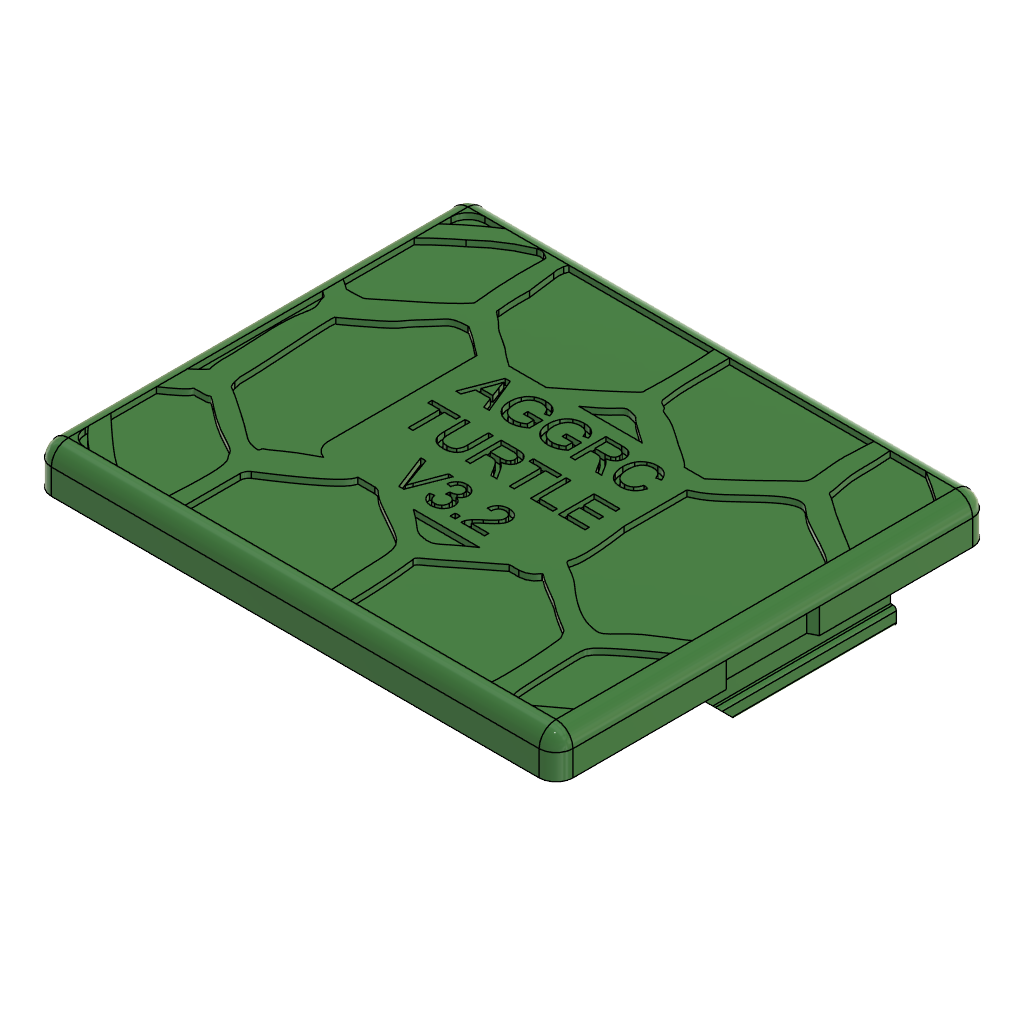
TURTLE_Case_TopV3 (Autodesk Fusion 360 design; units mm, degrees)
Autodesk Fusion 360 part; units mm, degrees
(part 1 of 2)
sketch "Sketch1" plane through (0, 0, 0) normal (0, 0, 1) x (1, 0, 0)
  line L0 (19.1, 22.9) -> (-19.1, 22.9) construction
  line L1 (-19.1, 22.9) -> (-19.1, -22.9) construction
  line L2 (19.1, -22.9) -> (19.1, 22.9) construction
  line L3 (19.1, 22.9) -> (-19.1, -22.9) construction
  line L4 (-19.1, 22.9) -> (19.1, -22.9) construction
  line L5 (18.1, -21.701) -> (18.1, -21.7) construction
  circle A0 centre (16.3, -20.1) radius 1.8 construction
  circle A1 centre (-16.3, -20.1) radius 1.8 construction
  line L6 (-7.8453, -9.4062) -> (-6.5, -9.4062) construction
  line L7 (-19.1, -22.9) -> (19.1, -22.9) construction
  line L8 (7.3, -22.9) -> (0.3, -22.9) construction
  line L9 (0.3, -22.9) -> (0.3, -10.4809) construction
  line L10 (0.3, -10.4809) -> (7.3, -10.4809) construction
  line L11 (7.3, -10.4809) -> (7.3, -22.9) construction
  line L12 (-11.4, -22.9) -> (-4.4, -22.9) construction
  line L13 (-4.4, -22.9) -> (-4.4, -10.4508) construction
  line L14 (-4.4, -10.4508) -> (-11.4, -10.4508) construction
  line L15 (-11.4, -10.4508) -> (-11.4, -22.9) construction
  line L16 (20.1, 22.9) -> (20.1, 23.7) construction
  line L17 (25.2, 25.2) -> (32.7, 25.2) construction
  line L18 (32.7, 25.2) -> (25.2, 25.2) construction
  line L19 (25.2, 25.2) -> (25.2, 16) construction
  line L20 (25.2, 16) -> (32.7, 16) construction
  line L21 (32.7, 16) -> (32.7, 25.2) construction
  line L22 (32.7, 25.2) -> (32.7, 23.7) construction
  line L23 (32.7, 23.7) -> (37.9, 23.7) construction
  line L24 (37.9, 23.7) -> (20.1, 23.7) construction
  line L25 (20.1, 23.7) -> (20.1, -19.5) construction
  line L26 (37.9, -19.5) -> (37.9, 23.7) construction
  line L27 (37.9, 23.7) -> (-19.1, 23.7) construction
  line L28 (-19.1, 23.7) -> (-19.1, -22.9) construction
  line L29 (-19.1, -22.9) -> (37.9, -22.9) construction
  line L30 (37.9, -22.9) -> (37.9, 23.7) construction
  line L31 (38.3, 24.1) -> (-19.5, 24.1) construction
  line L32 (-19.5, 24.1) -> (-19.5, -23.3) construction
  line L33 (-19.5, -23.3) -> (38.3, -23.3) construction
  line L34 (38.3, -23.3) -> (38.3, 24.1) construction
  line L35 (-19.5, 24.1) -> (38.3, 24.1)
  line L36 (38.3, 24.1) -> (38.3, -23.3)
  line L37 (38.3, -23.3) -> (-19.5, -23.3)
  line L38 (-19.5, -23.3) -> (-19.5, 24.1)
  line L39 (19.1, 22.9) -> (19.3, 22.9) construction
  line L40 (20.1, 22.9) -> (19.9, 22.9) construction
  line L41 (19.9, 23.7) -> (19.9, -23.3)
  line L42 (19.9, -23.3) -> (19.3, -23.3)
  line L43 (19.3, -23.3) -> (19.3, 23.7)
  line L44 (19.3, 23.7) -> (19.3, 24.1)
  line L45 (19.9, 23.7) -> (19.9, 24.1)
  circle A2 centre (-16.3, -20.1) radius 1.5
  circle A3 centre (16.3, -20.1) radius 1.5
  line L46 (25.2, 25.2) -> (25.2, 16) construction
  line L47 (16.7646, 20.1) -> (16.798, 20.1) construction
  circle A4 centre (16.6536, 20.4536) radius 1.5
  circle A5 centre (-16.5121, 20.3121) radius 1.5
  arc A6 (-17.5728, 21.3728) -> (-17.7041, 21.2263) centre (-16.3, 20.1) ccw construction
  line L48 (38.3, -19.9) -> (38.3, -19.4) construction
  line L49 (-14.9395, -20.1) -> (-14.9395, -20.6)
  line L50 (-14.9395, -20.1) -> (14.9498, -20.1)
  line L51 (14.9498, -20.1) -> (14.9498, -23.3)
  line L52 (14.9498, -23.3) -> (-14.9395, -23.3)
  line L53 (-14.9395, -23.3) -> (-14.9395, -20.1)
  line L54 (-14.9395, -20.6) -> (-14.5708, -20.6)
  line L55 (14.9498, -20.6) -> (14.9503, -20.6)
  line L56 (40.2, -25.2) -> (-21.4, -25.2)
  line L57 (-21.4, -25.2) -> (-21.4, 26)
  line L58 (-21.4, 26) -> (40.2, 26)
  line L59 (40.2, 26) -> (40.2, -25.2)
  line L60 (41.2, -26.2) -> (-22.4, -26.2)
  line L61 (-22.4, -26.2) -> (-22.4, 27)
  line L62 (-22.4, 27) -> (41.2, 27)
  line L63 (41.2, 27) -> (41.2, -26.2)
  line L64 (32.7, 24.0729) -> (25.2, 24.0729)
  line L65 (25.2, 24.0729) -> (25.2, 18.0729)
  line L66 (25.2, 18.0729) -> (32.7, 18.0729)
  line L67 (32.7, 18.0729) -> (32.7, 24.0729)
  line L68 (38.3, -19.65) -> (19.9, -19.65)
  line L69 (20.1, -19.4989) -> (19.9, -19.5)
  dimension "d1" = 38.2
  dimension "d2" = 45.8
  dimension "d5" = 3.6
  dimension "d7" = 2.8
  dimension "d13" = 7
  dimension "d14" = 11.8
  dimension "d15" = 7
  dimension "d16" = 7.7
  dimension "d17" = 1
  dimension "d23" = 7.5
  dimension "d24" = 9.2
  dimension "d25" = 1.5
  dimension "d26" = 5.2
  dimension "d27" = 17.8
  dimension "d28" = 43.2
  dimension "d31" = 0.4
  dimension "d36" = 0.2
  dimension "d37" = 0.2
  dimension "d54" = 3
  dimension "d57" = 3
  dimension "d67" = 3
  dimension "d69" = 0.3
  dimension "d70" = 3
  dimension "d89" = 0.5
  dimension "d237" = -1
  dimension "d283" = 6
  constraint horizontal L0
  constraint perpendicular L0 L1
  constraint parallel L1 L2
  constraint coincident L3 origin
  constraint coincident L4 origin
  constraint coincident L4 L5.start
  constraint horizontal L6
  constraint coincident L3 L6.start
  constraint perpendicular L2 L7
  constraint horizontal L8
  constraint vertical L9
  constraint horizontal L10
  constraint vertical L11
  constraint coincident L7 L8.start
  constraint horizontal L12
  constraint vertical L13
  constraint horizontal L14
  constraint vertical L15
  constraint coincident L7 L12.start
  constraint perpendicular L16 L17
  constraint horizontal L18
  constraint vertical L19
  constraint horizontal L20
  constraint vertical L21
  constraint perpendicular L17 L22
  constraint perpendicular L22 L23
  constraint horizontal L24
  constraint vertical L25
  constraint vertical L26
  constraint horizontal L27
  constraint vertical L28
  constraint horizontal L29
  constraint vertical L30
  constraint horizontal L35
  constraint vertical L36
  constraint horizontal L37
  constraint vertical L38
  constraint perpendicular L2 L39
  constraint perpendicular L16 L40
  constraint vertical L41
  constraint horizontal L42
  constraint vertical L43
  constraint coincident L37 L41.end
  constraint coincident L27 L43.end
  constraint coincident L35 L44.end
  constraint perpendicular L35 L44
  constraint coincident L31 L45.end
  constraint perpendicular L31 L45
  constraint concentric A0 A3
  constraint perpendicular L24 L46
  constraint coincident L34 L48.start
  constraint horizontal L47
  constraint coincident L3 L47.start
  constraint coincident A5 A6.start
  constraint coincident L4 A6.end
  constraint coincident L41 L69.end
  constraint perpendicular L49 L54
  constraint horizontal L50
  constraint vertical L51
  constraint horizontal L52
  constraint vertical L53
  constraint coincident L33 L51.end
  constraint coincident L51 L55.start
  constraint collinear L54 L55
  constraint coincident A1 L54.end
  constraint horizontal L64
  constraint vertical L65
  constraint horizontal L66
  constraint vertical L67
  constraint coincident L21 L64.start
  constraint midpoint L48 L68.start
  constraint coincident L41 L68.end
  constraint perpendicular L41 L68
  constraint coincident L25 L69.start
  measures "d1" distance of L1.end L2.start
  measures "d2" distance of L0.end L1.end
  measures "d5" diameter of A0
  measures "d7" distance of L2 A0.centre
  measures "d13" distance of L8.start L8.end
  measures "d14" distance of L2 L11
  measures "d15" distance of L12.start L12.end
  measures "d16" distance of L1 L15
  measures "d17" distance of L0.start L16.start
  measures "d23" distance of L17.end L17.start
  measures "d24" distance of L17.end L20.end
  measures "d25" distance of L17.end L22.end
  measures "d26" distance of L22.end L23.end
  measures "d27" distance of L23.end L16.end
  measures "d28" distance of L23.end L26.start
  measures "d36" distance of L0.start L39.end
  measures "d37" distance of L16.start L40.end
  measures "d54" diameter of A2
  measures "d57" diameter of A3
  measures "d67" diameter of A4
  measures "d69" distance of A6.centre A5.centre
  measures "d70" diameter of A5
  measures "d89" distance of L48.start L48.end
  measures "d283" distance of L64.start L66.end
extrude "Extrude1" add sketch "Sketch1" along normal blind 2 contours L35 L37 L38 L43 L44 A2 A3 L50 L51 L53 | L35 L37 L41 L42 L43 L44 L45 | L35 L36 L41 L45 L68 | L64 L65 L66 L67 makes body 1
extrude "Extrude2" add sketch "Sketch1" along normal blind 10.2 contours L36 L37 L41 L68 | L56 L57 L58 L59 bodies 1
extrude "Extrude16" add sketch "Sketch1" along normal blind 6 contours L37 A2 A3 L50 L51 L52 L53 bodies 1
extrude "Extrude3" add sketch "Sketch1" along normal blind 10 contours A2 L53 L54 | A2 L49 L50 L53 | A3 L50 L51 | A3 L50 L51 | A2 L49 L50 L53 L54 | A4 | A5 bodies 1
extrude "Extrude12" add sketch "Sketch1" along normal blind 16 contours L35 L37 L41 L42 L43 L44 L45 bodies 1
extrude "Extrude32" add sketch "Sketch1" along normal blind 6 contours L64 L65 L66 L67 bodies 1
ref_plane "WorkPlane1" through (9.4, 0.4, 10.2) normal (0, 0, 1) x (1, 0, 0)
sketch "Sketch3" plane through (0, 0, 10.2) normal (0, 0, 1) x (1, 0, 0)
  line L0 (25.2, 25.2) -> (25.2, 16)
  line L1 (32.7, 25.2) -> (25.2, 25.2)
  line L2 (32.7, 16) -> (32.7, 25.2)
  line L3 (25.2, 16) -> (32.7, 16)
  line L4 (25.2, 24.1) -> (24.9, 24.1) construction
  line L5 (32.7, 24.1) -> (33, 24.1) construction
  line L6 (24.9, 24.1) -> (33, 24.1)
  line L7 (33, 24.1) -> (33, 26)
  line L8 (24.9, 26) -> (24.9, 24.1)
  line L9 (0.3, -22.9) -> (0.3, -10.4809)
  line L10 (0.3, -10.4809) -> (7.3, -10.4809)
  line L11 (7.3, -10.4809) -> (7.3, -22.9)
  line L12 (-19.1, -22.9) -> (37.9, -22.9)
  line L13 (-4.4, -22.9) -> (-4.4, -10.4508)
  line L14 (-4.4, -10.4508) -> (-11.4, -10.4508)
  line L15 (-11.4, -10.4508) -> (-11.4, -22.9)
  line L16 (7.3, -22.9) -> (8, -22.9) construction
  line L17 (0.3, -22.9) -> (-0.4, -22.9) construction
  line L18 (-4.4, -22.9) -> (-3.7, -22.9) construction
  line L19 (8, -23.3) -> (8, -22.9)
  line L20 (-12.1, -22.9) -> (-12.1, -25.2)
  line L21 (-3.7, -25.2) -> (-3.7, -23.3)
  line L22 (-19.5, -23.3) -> (-19.5, 24.1)
  line L23 (-19.5, 24.1) -> (38.3, 24.1)
  line L24 (19.9, 23.7) -> (19.9, -23.3)
  line L25 (19.3, -23.3) -> (19.3, 23.7)
  line L26 (19.9, 23.7) -> (19.9, 24.1)
  line L27 (19.3, 23.7) -> (19.3, 24.1)
  line L28 (38.3, -23.3) -> (38.3, 24.1)
  line L29 (-19.5, -23.3) -> (38.3, -23.3)
  line L30 (19.9, -22.9) -> (38.3, -22.9)
  line L31 (38.3, -22.9) -> (38.3, -19.9)
  line L32 (19.9, -19.9) -> (19.9, -22.9)
  line L33 (38.3, 24.1) -> (38.3, -19.65)
  line L34 (19.9, -23.3) -> (19.3, -23.3)
  line L35 (24.9, 24.1) -> (33, 24.1)
  line L36 (33, 24.1) -> (33, 27)
  line L37 (33, 27) -> (24.9, 27)
  line L38 (24.9, 27) -> (24.9, 24.1)
  line L39 (-11.4, -22.9) -> (-3.6915, -22.9)
  line L40 (-3.6915, -26.2) -> (-12.1, -26.2)
  line L41 (-0.4, -22.9) -> (8.0023, -22.9)
  line L42 (8.0023, -23.3) -> (8.0023, -26.2)
  line L43 (8.0023, -26.2) -> (-0.4, -26.2)
  line L44 (-0.4, -26.2) -> (-0.4, -22.9)
  line L45 (-3.6915, -22.9) -> (-3.6915, -23.3)
  line L46 (-3.6915, -25.2) -> (-3.6915, -26.2)
  line L47 (-12.1, -26.2) -> (-12.1, -25.2)
  line L48 (-3.7, -22.9) -> (-4.4, -22.9)
  line L49 (-11.4, -22.9) -> (-12.1, -22.9)
  line L50 (8, -22.9) -> (7.3, -22.9)
  line L51 (0.3, -22.9) -> (-0.4, -22.9)
  line L52 (-3.6915, -22.9) -> (-12.1, -22.9)
  line L53 (-12.1, -22.9) -> (-12.1, -26.2)
  line L54 (-12.1, -26.2) -> (-3.6915, -26.2)
  line L55 (-3.6915, -26.2) -> (-3.6915, -22.9)
  line L56 (19.3, -23.3) -> (-19.5, -23.3)
  line L57 (-19.5, -23.3) -> (-19.5, 24.1)
  line L58 (-19.5, 24.1) -> (19.3, 24.1)
  line L59 (19.3, 24.1) -> (19.9, 24.1)
  line L60 (40.2, 26) -> (-21.4, 26)
  line L61 (-21.4, 26) -> (-21.4, -25.2)
  line L62 (-21.4, -25.2) -> (40.2, -25.2)
  line L63 (40.2, -25.2) -> (40.2, 26)
  line L64 (38.3, -19.65) -> (19.9, -19.65)
  line L65 (19.9, -19.65) -> (19.9, -23.3)
  line L66 (19.9, 24.1) -> (38.3, 24.1)
  dimension "d59" = 0.3
  dimension "d60" = 0.3
  dimension "d71" = 0.7
  dimension "d72" = 0.7
  dimension "d73" = 0.7
  constraint coincident L0 L4.start
  constraint perpendicular L0 L4
  constraint coincident L2 L5.start
  constraint perpendicular L2 L5
  constraint perpendicular L6 L7
  constraint parallel L7 L8
  constraint perpendicular L2 L6
  constraint coincident L11.end L16.start
  constraint perpendicular L11 L16
  constraint coincident L9.start L17.start
  constraint perpendicular L9 L17
  constraint coincident L13.start L18.start
  constraint perpendicular L13 L18
  constraint horizontal L50
  constraint vertical L19
  constraint horizontal L48
  constraint vertical L20
  constraint vertical L21
  constraint horizontal L30
  constraint vertical L31
  constraint vertical L32
  constraint coincident L24 L30.start
  constraint coincident L12 L30.start
  constraint horizontal L35
  constraint vertical L36
  constraint horizontal L37
  constraint vertical L38
  constraint horizontal L39
  constraint vertical L45
  constraint horizontal L40
  constraint vertical L47
  constraint horizontal L41
  constraint vertical L42
  constraint horizontal L43
  constraint vertical L44
  constraint coincident L29 L21.end
  constraint coincident L29 L45.end
  constraint collinear L45 L46
  constraint collinear L48 L49
  constraint collinear L50 L51
  constraint coincident L29 L19.start
  constraint coincident L29 L42.start
  constraint horizontal L52
  constraint vertical L53
  constraint horizontal L54
  constraint vertical L55
  measures "d59" distance of L4.start L4.end
  measures "d60" distance of L5.start L5.end
  measures "d71" distance of L11.end L16.end
  measures "d72" distance of L9.start L17.end
  measures "d73" distance of L13.start L18.end
extrude "Extrude5" cut sketch "Sketch3" against normal blind 3.9 contours L0 L1 L2 L6 L23 L35 L66 | L0 L1 L2 L6 L7 L8 L23 L35 L36 L38 L60 L66 | L36 L37 L38 L60 | L40 L46 L47 L53 L54 L55 L62 | L20 L21 L29 L53 L56 L62 | L29 L42 L44 L56 L62 | L42 L43 L44 L62 | L12 L20 L29 L39 L45 L48 L49 L52 L53 L55 L56 | L21 L29 L55 L56 L62 | L12 L19 L29 L41 L44 L50 L51 L56 bodies 1
extrude "Extrude13" add sketch "Sketch3" along normal blind 14.2 contours L0 L1 L2 L6 L23 L35 L66 | L0 L1 L2 L6 L7 L8 L23 L35 L36 L38 L60 L66 | L8 L20 L22 L23 L29 L38 L53 L56 L57 L58 L59 L60 L61 L62 L66 | L7 L23 L28 L29 L31 L33 L34 L36 L42 L56 L60 L62 L63 L66 | L29 L44 L55 L56 L62 bodies 1
sketch "Sketch10" plane through (0, 0, 24.4) normal (0, 0, 1) x (-1, 0, 0)
  line L0 (19.5, -24.1) -> (-38.3, -24.1)
  line L1 (3.6915, 23.3) -> (12.1, 23.3)
  line L2 (12.1, 23.3) -> (12.1, 25.2)
  line L3 (3.6915, 25.2) -> (3.6915, 23.3)
  line L4 (0.4, 25.2) -> (0.4, 23.3)
  line L5 (0.4, 23.3) -> (3.6915, 23.3)
  line L6 (3.6915, 23.3) -> (3.6915, 25.2)
  line L7 (-8.0023, 23.3) -> (0.4, 23.3)
  line L8 (0.4, 23.3) -> (0.4, 25.2)
  line L9 (-8.0023, 25.2) -> (-8.0023, 23.3)
  line L10 (12.1, 23.3) -> (19.5, 23.3)
  line L11 (19.5, 23.3) -> (19.5, -24.1)
  line L12 (-38.3, -24.1) -> (-38.3, 23.3)
  line L13 (-38.3, 23.3) -> (-8.0023, 23.3)
  line L14 (-8.0023, 23.3) -> (-8.0023, 25.2)
  line L15 (-8.0023, 25.2) -> (-40.2, 25.2)
  line L16 (-40.2, 25.2) -> (-40.2, -26)
  line L17 (-40.2, -26) -> (21.4, -26)
  line L18 (21.4, -26) -> (21.4, 25.2)
  line L19 (21.4, 25.2) -> (12.1, 25.2)
  line L20 (12.1, 25.2) -> (12.1, 23.3)
  line L21 (12.1, 25.2) -> (3.6915, 25.2)
  line L22 (3.6915, 25.2) -> (0.4, 25.2)
  line L23 (0.4, 25.2) -> (-8.0023, 25.2)
extrude "Extrude22" add sketch "Sketch10" along normal blind 7 contours L0 L2 L9 L10 L11 L12 L13 L14 L15 L16 L17 L18 L19 L20 | L1 L2 L3 L6 L20 L21 | L4 L7 L8 L9 L14 L23 | L3 L4 L5 L6 L8 L22 bodies 1
sketch "Sketch13" plane through (0, 0, 31.4) normal (0, 0, 1) x (-1, 0, 0)
  line L0 (-38.3, 23.3) -> (19.5, 23.3)
  line L1 (-7.9258, 23.3) -> (-7.9258, 23.1) construction
  line L2 (-38.3, 23.3) -> (-38.3, -0.4) construction
  line L3 (19.5, 23.3) -> (19.5, -0.4) construction
  line L4 (-38.3, -0.4) -> (-38.3, 17.6) construction
  line L5 (-38.3, -0.4) -> (-38.3, -18.4) construction
  line L6 (19.5, -0.4) -> (19.5, 17.6) construction
  line L7 (19.5, -0.4) -> (19.5, -18.4) construction
  line L8 (19.5, 17.6) -> (18.5, 17.6) construction
  line L9 (19.5, 17.6) -> (18.5, 17.6)
  line L10 (19.5, -18.4) -> (19.3, -18.4)
  line L11 (19.3, -18.4) -> (18.3, -18.4)
  line L12 (18.3, -18.4) -> (19.3, -18.4)
  line L13 (19.3, 17.6) -> (18.3, 17.6)
  line L14 (19.5, 23.3) -> (19.5, -24.1)
  line L15 (19.5, -24.1) -> (-38.3, -24.1)
  line L16 (-38.3, -24.1) -> (-38.3, 23.3)
  line L17 (21.4, 25.2) -> (-40.2, 25.2)
  line L18 (-40.2, 25.2) -> (-40.2, -26)
  line L19 (-40.2, -26) -> (21.4, -26)
  line L20 (21.4, -26) -> (21.4, 25.2)
  line L21 (-37.1, 10.6) -> (-38.1, 10.6) construction
  line L22 (-37.1, -16.4) -> (-37.1, 10.6)
  line L23 (-37.1, 10.6) -> (-38.1, 10.6)
  line L24 (-38.1, 10.6) -> (-38.1, -16.4)
  line L25 (-38.1, -16.4) -> (-37.1, -16.4)
  line L26 (-38.1, -16.4) -> (-38.3, -16.4)
  line L27 (-38.3, -16.4) -> (-38.3, 10.6)
  line L28 (-38.3, 10.6) -> (-38.1, 10.6)
  line L29 (19.3, -18.4) -> (19.5, -18.4)
  line L30 (19.5, -18.4) -> (19.5, 17.6)
  line L31 (19.5, 17.6) -> (19.3, 17.6)
  line L32 (19.3, 17.6) -> (19.3, -18.4)
  line L33 (18.3, 17.6) -> (18.3, -18.4)
  line L34 (19.3, 17.6) -> (19.3, -18.4)
  line L35 (-38.1, -16.4) -> (-38.1, 10.6)
  line L36 (18.3, -22.9) -> (-37.1, -22.9)
  line L37 (-37.1, 22.1) -> (18.3, 22.1)
  line L38 (18.3, 17.6) -> (18.3, -18.4)
  line L39 (19.3, 17.6) -> (19.3, -18.4)
  line L40 (-37.1, -16.4) -> (-37.1, 10.6)
  line L41 (-38.1, -16.4) -> (-38.1, 10.6)
  line L42 (18.3, 22.1) -> (19.5, 22.1)
  line L43 (-37.1, 22.1) -> (-38.3, 22.1)
  line L44 (18.3, -22.9) -> (19.5, -22.9)
  line L45 (-37.1, -22.9) -> (-38.3, -22.9)
  dimension "d189" = 0.2
  dimension "d192" = 23.7
  dimension "d193" = 23.7
  dimension "d194" = 18
  dimension "d195" = 18
  dimension "d196" = 18
  dimension "d197" = 18
  dimension "d199" = 1
  constraint coincident L0 L1.start
  constraint coincident L0.start L2.start
  constraint perpendicular L0 L2
  constraint coincident L0.end L3.start
  constraint perpendicular L0 L3
  constraint parallel L2 L4
  constraint parallel L3 L6
  constraint perpendicular L3 L8
  constraint perpendicular L7 L10
  constraint perpendicular L7 L11
  constraint parallel L12 L13
  constraint perpendicular L22 L23
  constraint parallel L22 L24
  constraint parallel L23 L25
  constraint perpendicular L21 L22
  constraint horizontal L26
  constraint vertical L27
  constraint horizontal L28
  constraint coincident L16 L27.end
  constraint horizontal L29
  constraint vertical L30
  constraint horizontal L31
  constraint vertical L32
  constraint coincident L3 L42.end
  constraint coincident L2 L43.end
  constraint coincident L14 L44.end
  constraint perpendicular L14 L44
  constraint coincident L16 L45.end
  constraint perpendicular L16 L45
  measures "d189" distance of L1.start L1.end
  measures "d192" distance of L0.start L2.end
  measures "d193" distance of L0.end L3.end
  measures "d194" distance of L2.end L4.end
  measures "d195" distance of L2.end L5.end
  measures "d196" distance of L3.end L6.end
  measures "d197" distance of L3.end L7.end
  measures "d199" distance of L6.end L8.end
extrude "Extrude23" add sketch "Sketch13" along normal blind 5 separate body contours L0 L14 L16 L37 L42 L43 | L9 L10 L11 L12 L13 L14 L16 L22 L23 L25 L26 L28 L29 L31 L33 L36 L37 L38 L40 L42 L43 L44 L45 | L16 L24 L26 L27 L28 L35 L41 | L9 L10 L14 L29 L30 L31 L32 L34 L39 | L22 L23 L24 L25 L35 L40 L41 | L9 L11 L12 L13 L32 L33 L34 L38 L39 | L14 L15 L16 L36 L44 L45 | L17 L18 L19 L20 makes body 2
extrude "Extrude25" add sketch "Sketch13" against normal blind 5 contours L22 L23 L24 L25 L35 L40 L41 | L9 L11 L12 L13 L32 L33 L34 L38 L39 bodies 2
ref_plane "WorkPlane2" through (9.4, 0.4, 33.9) normal (1, 0, 0) x (0, 1, 0)
sketch "Sketch19" plane through (38.1, 0, 0) normal (1, 0, 0) x (0, 1, 0)
  line L0 (-10.6, 26.4) -> (16.4, 26.4)
  line L1 (16.4, 26.4) -> (-10.6, 26.4)
  line L2 (-10.6, 26.4) -> (-10.6, 28.4)
  line L3 (-10.6, 28.4) -> (16.4, 28.4)
  line L4 (16.4, 28.4) -> (16.4, 26.4)
  line L5 (16.4, 31.4) -> (-10.6, 31.4)
  line L6 (-10.6, 31.4) -> (-10.6, 26.4)
  line L7 (16.4, 26.4) -> (16.4, 31.4)
  dimension "d269" = 2
  constraint perpendicular L1 L2
  constraint parallel L1 L3
  constraint parallel L2 L4
  constraint coincident L0.start L1.end
  constraint coincident L0.end L1.start
  measures "d269" distance of L0.end L3.end
sketch "Sketch26" plane through (-19.3, 0, 0) normal (-1, 0, 0) x (0, -1, 0)
  line L0 (17.6, 31.4) -> (-18.4, 31.4)
  line L1 (-18.4, 31.4) -> (-18.4, 26.4)
  line L2 (-18.4, 26.4) -> (17.6, 26.4)
  line L3 (17.6, 26.4) -> (17.6, 31.4)
  line L4 (17.6, 26.4) -> (-18.4023, 26.4)
  line L5 (-18.4023, 26.4) -> (-18.4023, 28.4)
  line L6 (-18.4023, 28.4) -> (17.6, 28.4)
  line L7 (17.6, 28.4) -> (17.6, 26.4)
  dimension "d327" = 2
  constraint horizontal L4
  constraint vertical L5
  constraint horizontal L6
  constraint vertical L7
  constraint coincident L2.end L3.start
  measures "d327" distance of L2.end L6.end
extrude "Extrude27" add sketch "Sketch26" along normal blind 0.7 contours L1 L2 L3 L4 L6 L7 bodies 2
extrude "Extrude31" add sketch "Sketch19" along normal blind 0.7 contours L0 L1 L2 L3 L4 L6 L7 bodies 2
sketch "Sketch18" plane through (40.2, 0, 0) normal (1, 0, 0) x (0, 1, 0)
  line L0 (-25.2, 31.4) -> (26, 31.4)
  line L1 (26, 31.4) -> (26, 36.4)
  line L2 (26, 36.4) -> (-25.2, 36.4)
  line L3 (-25.2, 36.4) -> (-25.2, 31.4)
  line L4 (-25.2, 31.4) -> (0.4, 31.4) construction
  line L5 (0.4, 31.4) -> (5.4, 31.4) construction
  line L6 (0.4, 31.4) -> (-4.6, 31.4) construction
  line L7 (-4.6, 31.4) -> (5.4, 31.4)
  line L8 (5.4, 31.4) -> (5.4, 33.9)
  line L9 (5.4, 33.9) -> (-4.6, 33.9)
  line L10 (-4.6, 33.9) -> (-4.6, 31.4)
  dimension "d257" = 25.6
  dimension "d258" = 5
  dimension "d259" = 5
  dimension "d260" = 10
  dimension "d261" = 2.5
  constraint coincident L0.start L3.end
  constraint perpendicular L3 L4
  constraint coincident L0 L5.end
  constraint parallel L4 L6
  constraint horizontal L7
  constraint vertical L8
  constraint horizontal L9
  constraint vertical L10
  measures "d257" distance of L0.start L4.end
  measures "d258" distance of L4.end L5.end
  measures "d259" distance of L4.end L6.end
  measures "d260" distance of L6.end L5.end
  measures "d261" distance of L6.end L9.end
extrude "Extrude30" cut sketch "Sketch18" against normal blind 1 contours L0 L7 L8 L9 L10 bodies 2
mirror "Mirror2" about plane through (9.4, 0.4, 33.9) normal (1, 0, 0) of "Extrude30"
sketch "Sketch16" plane through (-19.5, 0, 0) normal (1, 0, 0) x (0, 1, 0)
  line L0 (-23.3, 2) -> (24.1, 2)
  line L1 (24.1, 2) -> (24.1, 31.4)
  line L2 (24.1, 31.4) -> (-23.3, 31.4)
  line L3 (-23.3, 31.4) -> (-23.3, 2)
  line L4 (-23.3, 31.4) -> (0.4, 31.4) construction
  line L5 (0.4, 31.4) -> (0.4, 28.4) construction
  line L6 (0.4, 28.4) -> (0.4, 26.4) construction
  line L7 (0.4, 26.4) -> (18.4, 26.4) construction
  line L8 (0.4, 26.4) -> (-17.6, 26.4) construction
  line L9 (-17.6, 26.4) -> (-17.6, 28.4) construction
  line L10 (-17.6, 28.4) -> (-17.6, 26.4)
  line L11 (-17.6, 26.4) -> (18.4, 26.4)
  line L12 (18.4, 26.4) -> (18.4, 28.4)
  line L13 (18.4, 28.4) -> (-17.6, 28.4)
  dimension "d222" = 23.7
  dimension "d223" = 3
  dimension "d224" = 2
  dimension "d225" = 18
  dimension "d226" = 18
  dimension "d227" = 2
  constraint coincident L2.end L3.start
  constraint midpoint L2 L4.end
  constraint perpendicular L4 L5
  constraint perpendicular L2 L6
  constraint perpendicular L6 L7
  constraint perpendicular L6 L8
  constraint perpendicular L8 L9
  constraint perpendicular L10 L11
  constraint parallel L10 L12
  constraint parallel L11 L13
  measures "d222" distance of L2.end L4.end
  measures "d223" distance of L4.end L5.end
  measures "d224" distance of L5.end L6.end
  measures "d225" distance of L6.end L7.end
  measures "d226" distance of L6.end L8.end
  measures "d227" distance of L8.end L9.end
extrude "Extrude28" cut sketch "Sketch16" against normal blind 0.7 contours L10 L11 L12 L13 bodies 1
extrude "Extrude29" cut sketch "Sketch13" along normal blind 3 contours L9 L10 L11 L12 L13 L14 L16 L22 L23 L25 L26 L28 L29 L31 L33 L36 L37 L38 L40 L42 L43 L44 L45 | L9 L10 L14 L29 L30 L31 L32 L34 L39 bodies 2
extrude "Extrude35" add sketch "Sketch13" against normal blind 2 contours L0 L14 L16 L37 L42 L43 | L14 L15 L16 L36 L44 L45 bodies 2
mirror "Mirror3" about plane through (9.4, 0.4, 33.9) normal (1, 0, 0) of "Extrude28"
sketch "Sketch17" plane through (9.4, 0, 0) normal (1, 0, 0) x (0, 1, 0)
fillet "Fillet16" radius 2 8 edges at (40.2, -25.2, 15.7) (40.2, 26, 15.7) (-21.4, 26, 15.7) (-21.4, -25.2, 15.7) (40.2, -25.2, 33.9) (40.2, 26, 33.9) (-21.4, 26, 33.9) (-21.4, -25.2, 33.9) on bodies 1 2
sketch "Sketch24" plane through (0, 0, 36.4) normal (0, 0, 1) x (-1, 0, 0)
  arc A0 (21.4, 23.2) -> (19.4, 25.2) centre (19.4, 23.2) ccw
  line L0 (19.4, 25.2) -> (-38.2, 25.2)
  arc A1 (-38.2, 25.2) -> (-40.2, 23.2) centre (-38.2, 23.2) ccw
  line L1 (-40.2, 23.2) -> (-40.2, -24)
  arc A2 (-40.2, -24) -> (-38.2, -26) centre (-38.2, -24) ccw
  line L2 (-38.2, -26) -> (19.4, -26)
  arc A3 (19.4, -26) -> (21.4, -24) centre (19.4, -24) ccw
  line L3 (21.4, -24) -> (21.4, 23.2)
  arc A4 (11.3811, -26) -> (21.4, -18.5141) centre (-2.7859, 3.4081) ccw
  arc A5 (11.0665, -23.7947) -> (16.1393, -20.5124) centre (4.942, -8.7683) ccw
  arc A6 (16.1393, -20.5124) -> (21.4, -15.4127) centre (-2.5631, 4.0438) ccw
  arc A7 (21.4, -15.4127) -> (21.4062, -15.4048) centre (-2.7344, 3.4965) ccw
  arc A8 (8.8605, -25.5305) -> (10.472, -26) centre (19.6633, 8.5476) ccw
  arc A9 (8.8605, -25.5305) -> (8.7, -26) centre (25.0805, -31.338) ccw
  arc A10 (9.6, -23.4) -> (10.2246, -23.7543) centre (15.2927, -14.0914) ccw
  arc A11 (9.534, -23.0852) -> (9.6, -23.4) centre (10.4467, -23.0583) ccw
  arc A12 (9.534, -23.0852) -> (9.2, -14.6) centre (-44.1135, -20.948) ccw
  arc A13 (6.7, -26) -> (7.63, -23.5408) centre (-18.1541, -15.1955) ccw
  arc A14 (7.63, -23.5408) -> (7.6141, -22.3338) centre (4.9418, -22.9727) ccw
  arc A15 (7.6141, -22.3338) -> (7.1948, -19.0652) centre (-155.4891, -41.592) ccw
  arc A16 (7.1948, -19.0652) -> (7.051, -15.2896) centre (-16.615, -18.0816) ccw
  spline S0 degree 5 poles (7.051, -15.2896) (7.056, -15.2681) (7.0638, -15.2264) (7.0693, -15.1681) (7.0642, -15.0984) (7.0334, -15.0211) (6.965, -14.9397) (6.8434, -14.8362) (6.663, -14.6984) (6.4379, -14.5288) (6.1934, -14.339) (5.9569, -14.144) (5.7497, -13.9575) (5.577, -13.7857) (5.4227, -13.6239) (5.2604, -13.4619) (5.0629, -13.2884) (4.811, -13.0949) (4.5046, -12.8813) (4.1592, -12.6543) (3.799, -12.4242) (3.4516, -12.2026) (3.1413, -11.9995) (2.8837, -11.821) (2.6785, -11.6657) (2.5088, -11.525) (2.3502, -11.387) (2.1774, -11.2394) (1.9719, -11.0738) (1.7286, -10.8878) (1.4515, -10.684) (1.1516, -10.4689) (0.843, -10.251) (0.5404, -10.0402) (0.2559, -9.8465) (-0.0031, -9.6785) (-0.2341, -9.543) (-0.4394, -9.4442) (-0.6267, -9.3828) (-0.8101, -9.3553) (-1.0069, -9.354) (-1.2306, -9.3694) (-1.4853, -9.3915) (-1.7575, -9.4119) (-2.0224, -9.4246) (-2.2554, -9.4286) (-2.4407, -9.4281) (-2.5844, -9.4358) (-2.7154, -9.4706) (-2.8696, -9.5519) (-3.0759, -9.6925) (-3.3462, -9.8951) (-3.6809, -10.1551) (-4.0709, -10.4623) (-4.5013, -10.8032) (-4.9538, -11.163) (-5.4107, -11.5278) (-5.8568, -11.8863) (-6.284, -12.2325) (-6.6894, -12.5648) (-7.0743, -12.8845) (-7.4421, -13.1944) (-7.7971, -13.4979) (-8.1424, -13.797) (-8.4783, -14.0917) (-8.8014, -14.3781) (-9.1015, -14.6469) (-9.3643, -14.8855) (-9.5756, -15.082) (-9.7254, -15.23) (-9.8115, -15.3312) (-9.8452, -15.4017) (-9.85, -15.4705) (-9.8472, -15.5672) (-9.8463, -15.7131) (-9.8499, -15.9228) (-9.8573, -16.2034) (-9.8673, -16.5559) (-9.8784, -16.9759) (-9.8891, -17.4552) (-9.8977, -17.9826) (-9.9028, -18.5451) (-9.9031, -19.1294) (-9.8978, -19.7229) (-9.8866, -20.315) (-9.8697, -20.8973) (-9.8477, -21.4634) (-9.8218, -22.0089) (-9.7931, -22.5306) (-9.763, -23.0263) (-9.7329, -23.4952) (-9.704, -23.9367) (-9.6774, -24.3506) (-9.6539, -24.737) (-9.6341, -25.0958) (-9.6183, -25.4271) (-9.6089, -25.67) (-9.6037, -25.8398) (-9.6011, -25.9475) (-9.6, -26) knots 0 0 0 0 0 0 0.01052632 0.02105263 0.03157895 0.04210526 0.05263158 0.06315789 0.07368421 0.08421053 0.09473684 0.10526316 0.11578947 0.12631579 0.13684211 0.14736842 0.15789474 0.16842105 0.17894737 0.18947368 0.2 0.21052632 0.22105263 0.23157895 0.24210526 0.25263158 0.26315789 0.27368421 0.28421053 0.29473684 0.30526316 0.31578947 0.32631579 0.33684211 0.34736842 0.35789474 0.36842105 0.37894737 0.38947368 0.4 0.41052632 0.42105263 0.43157895 0.44210526 0.45263158 0.46315789 0.47368421 0.48421053 0.49473684 0.50526316 0.51578947 0.52631579 0.53684211 0.54736842 0.55789474 0.56842105 0.57894737 0.58947368 0.6 0.61052632 0.62105263 0.63157895 0.64210526 0.65263158 0.66315789 0.67368421 0.68421053 0.69473684 0.70526316 0.71578947 0.72631579 0.73684211 0.74736842 0.75789474 0.76842105 0.77894737 0.78947368 0.8 0.81052632 0.82105263 0.83157895 0.84210526 0.85263158 0.86315789 0.87368421 0.88421053 0.89473684 0.90526316 0.91578947 0.92631579 0.93684211 0.94736842 0.95789474 0.96842105 0.97894737 0.98947368 1 1 1 1 1 1
  spline S1 degree 5 poles (21.4, -10.5) (21.3681, -10.4783) (21.3002, -10.4327) (21.1856, -10.3574) (21.0075, -10.2433) (20.7436, -10.0782) (20.4417, -9.8923) (20.1082, -9.6886) (19.7541, -9.4723) (19.3961, -9.2516) (19.0571, -9.0373) (18.7606, -8.8415) (18.5251, -8.6755) (18.3587, -8.5476) (18.2547, -8.4619) (18.1829, -8.4153) (18.095, -8.3982) (17.9463, -8.3987) (17.7197, -8.4076) (17.4328, -8.4195) (17.1209, -8.432) (16.8267, -8.444) (16.5871, -8.4551) (16.4191, -8.4637) (16.3158, -8.4685) (16.2553, -8.4714) (16.207, -8.4822) (16.1388, -8.5197) (16.0222, -8.6038) (15.8405, -8.7465) (15.5894, -8.9491) (15.2741, -9.2057) (14.9066, -9.505) (14.5031, -9.8328) (14.081, -10.1741) (13.6569, -10.5154) (13.2429, -10.8471) (12.8459, -11.1649) (12.4685, -11.4683) (12.1103, -11.7593) (11.769, -12.0415) (11.4413, -12.3193) (11.1244, -12.5961) (10.8167, -12.8738) (10.519, -13.1515) (10.2356, -13.4245) (9.9725, -13.6862) (9.7369, -13.9285) (9.5363, -14.1432) (9.3774, -14.323) (9.265, -14.4623) (9.2142, -14.5393) (9.1984, -14.5773) (9.1978, -14.5939) (9.2, -14.6) knots 0 0 0 0 0 0 0.02 0.04 0.06 0.08 0.1 0.12 0.14 0.16 0.18 0.2 0.22 0.24 0.26 0.28 0.3 0.32 0.34 0.36 0.38 0.4 0.42 0.44 0.46 0.48 0.5 0.52 0.54 0.56 0.58 0.6 0.62 0.64 0.66 0.68 0.7 0.72 0.74 0.76 0.78 0.8 0.82 0.84 0.86 0.88 0.9 0.92 0.94 0.96 0.98 1 1 1 1 1 1
  arc A17 (10.2246, -23.7543) -> (11.0665, -23.7947) centre (10.6891, -22.8687) ccw
  spline S2 degree 5 poles (21.4, -7.9) (21.3016, -7.8554) (21.1096, -7.7673) (20.8363, -7.6383) (20.5015, -7.4726) (20.1321, -7.2765) (19.8113, -7.0921) (19.5381, -6.921) (19.3111, -6.7658) (19.1278, -6.6304) (18.9846, -6.5204) (18.8769, -6.4427) (18.7991, -6.3979) (18.745, -6.3733) (18.708, -6.335) (18.6801, -6.2479) (18.6506, -6.1044) (18.6082, -5.9207) (18.5451, -5.7215) (18.4608, -5.526) (18.3654, -5.3367) (18.2738, -5.1463) (18.2015, -4.9434) (18.1607, -4.7177) (18.1542, -4.4663) (18.1779, -4.193) (18.223, -3.9049) (18.2788, -3.6106) (18.3353, -3.3176) (18.3857, -3.0295) (18.4272, -2.7461) (18.4594, -2.4639) (18.4838, -2.1776) (18.5023, -1.8806) (18.5168, -1.5659) (18.5277, -1.2272) (18.535, -0.8589) (18.5379, -0.4572) (18.5354, -0.02) (18.5266, 0.4525) (18.5109, 0.9569) (18.4886, 1.487) (18.4605, 2.0322) (18.4287, 2.5789) (18.3957, 3.112) (18.3643, 3.6166) (18.3371, 4.0794) (18.3163, 4.491) (18.3032, 4.8466) (18.298, 5.1485) (18.2995, 5.4074) (18.3048, 5.6435) (18.3097, 5.88) (18.31, 6.1368) (18.3015, 6.425) (18.281, 6.7403) (18.2468, 7.058) (18.2, 7.3455) (18.1456, 7.5727) (18.0933, 7.723) (18.0589, 7.8051) (18.0651, 7.8621) (18.1311, 7.944) (18.2604, 8.077) (18.441, 8.2574) (18.6526, 8.4663) (18.8733, 8.6781) (19.085, 8.8699) (19.2807, 9.0332) (19.4628, 9.1708) (19.6389, 9.2928) (19.8196, 9.4129) (20.0153, 9.544) (20.2329, 9.6953) (20.4772, 9.873) (20.7511, 10.0807) (20.995, 10.2722) (21.192, 10.4305) (21.3296, 10.5424) (21.4, 10.6) knots 0 0 0 0 0 0 0.01333333 0.02666667 0.04 0.05333333 0.06666667 0.08 0.09333333 0.10666667 0.12 0.13333333 0.14666667 0.16 0.17333333 0.18666667 0.2 0.21333333 0.22666667 0.24 0.25333333 0.26666667 0.28 0.29333333 0.30666667 0.32 0.33333333 0.34666667 0.36 0.37333333 0.38666667 0.4 0.41333333 0.42666667 0.44 0.45333333 0.46666667 0.48 0.49333333 0.50666667 0.52 0.53333333 0.54666667 0.56 0.57333333 0.58666667 0.6 0.61333333 0.62666667 0.64 0.65333333 0.66666667 0.68 0.69333333 0.70666667 0.72 0.73333333 0.74666667 0.76 0.77333333 0.78666667 0.8 0.81333333 0.82666667 0.84 0.85333333 0.86666667 0.88 0.89333333 0.90666667 0.92 0.93333333 0.94666667 0.96 0.97333333 0.98666667 1 1 1 1 1 1
  spline S3 degree 5 poles (15.9, -4.9) (15.8317, -4.9488) (15.6932, -5.0481) (15.4802, -5.2022) (15.1854, -5.4179) (14.7996, -5.7042) (14.3985, -6.0059) (13.9862, -6.3205) (13.57, -6.6434) (13.1605, -6.9675) (12.7734, -7.2829) (12.426, -7.5784) (12.1329, -7.8446) (11.9021, -8.0764) (11.7315, -8.2758) (11.6033, -8.4548) (11.4848, -8.6353) (11.3415, -8.8403) (11.1459, -9.0878) (10.8911, -9.3819) (10.5914, -9.7116) (10.2725, -10.0578) (9.9642, -10.397) (9.6914, -10.7074) (9.4666, -10.9729) (9.2815, -11.1893) (9.114, -11.3597) (8.9359, -11.492) (8.72, -11.595) (8.4482, -11.6749) (8.11, -11.7353) (7.7823, -11.7696) (7.5039, -11.7877) (7.3037, -11.7965) (7.2, -11.8) knots 0 0 0 0 0 0 0.033333 0.066667 0.1 0.133333 0.166667 0.2 0.233333 0.266667 0.3 0.333333 0.366667 0.4 0.433333 0.466667 0.5 0.533333 0.566667 0.6 0.633333 0.666667 0.7 0.733333 0.766667 0.8 0.833333 0.866667 0.9 0.933333 0.966667 1 1 1 1 1 1
  spline S4 degree 5 poles (7.2, -11.8) (7.1942, -11.8029) (7.1821, -11.8075) (7.1623, -11.8114) (7.1327, -11.8103) (7.0905, -11.7987) (7.044, -11.7776) (6.9946, -11.7483) (6.9429, -11.712) (6.8879, -11.6696) (6.8254, -11.6213) (6.7511, -11.5666) (6.6612, -11.5054) (6.5556, -11.4377) (6.4367, -11.3642) (6.3082, -11.2853) (6.174, -11.2011) (6.0361, -11.1109) (5.8939, -11.0131) (5.7448, -10.9056) (5.5854, -10.7859) (5.4119, -10.6521) (5.2211, -10.5031) (5.0119, -10.3392) (4.7849, -10.1623) (4.5428, -9.9754) (4.2892, -9.7823) (4.0283, -9.5873) (3.7644, -9.3943) (3.5015, -9.2068) (3.2424, -9.0274) (2.9888, -8.8574) (2.74, -8.6959) (2.4938, -8.5409) (2.2474, -8.3895) (1.9976, -8.2385) (1.7419, -8.0852) (1.479, -7.9278) (1.2096, -7.766) (0.9369, -7.6018) (0.6676, -7.4398) (0.4112, -7.287) (0.1783, -7.1512) (-0.0213, -7.0392) (-0.18, -6.9555) (-0.2942, -6.9011) (-0.3658, -6.8719) (-0.4042, -6.8566) (-0.4231, -6.8406) (-0.4368, -6.8106) (-0.455, -6.7593) (-0.4843, -6.6838) (-0.5286, -6.584) (-0.5908, -6.4602) (-0.6725, -6.3125) (-0.7748, -6.141) (-0.8736, -5.9848) (-0.9573, -5.857) (-1.0173, -5.767) (-1.0484, -5.7209) knots 0 0 0 0 0 0 0.018182 0.036364 0.054545 0.072727 0.090909 0.109091 0.127273 0.145455 0.163636 0.181818 0.2 0.218182 0.236364 0.254545 0.272727 0.290909 0.309091 0.327273 0.345455 0.363636 0.381818 0.4 0.418182 0.436364 0.454545 0.472727 0.490909 0.509091 0.527273 0.545455 0.563636 0.581818 0.6 0.618182 0.636364 0.654545 0.672727 0.690909 0.709091 0.727273 0.745455 0.763636 0.781818 0.8 0.818182 0.836364 0.854545 0.872727 0.890909 0.909091 0.927273 0.945455 0.963636 0.981818 1 1 1 1 1 1
  spline S5 degree 5 poles (-1.0484, -5.7209) (-1.0555, -5.7153) (-1.0686, -5.704) (-1.0848, -5.6867) (-1.0994, -5.6631) (-1.1062, -5.6325) (-1.1023, -5.6006) (-1.0894, -5.5671) (-1.0708, -5.5314) (-1.0502, -5.4924) (-1.0312, -5.4485) (-1.0165, -5.3973) (-1.007, -5.3353) (-1.0021, -5.2584) (-1.0004, -5.1623) (-1, -5.0432) (-0.9992, -4.898) (-0.9969, -4.7249) (-0.9921, -4.5231) (-0.9846, -4.2924) (-0.9739, -4.033) (-0.9628, -3.8028) (-0.953, -3.6176) (-0.9458, -3.4886) (-0.9421, -3.4226) knots 0 0 0 0 0 0 0.05 0.1 0.15 0.2 0.25 0.3 0.35 0.4 0.45 0.5 0.55 0.6 0.65 0.7 0.75 0.8 0.85 0.9 0.95 1 1 1 1 1 1
  spline S6 degree 5 poles (-0.9421, -3.4226) (-0.9495, -3.2501) (-0.9646, -2.9087) (-0.9884, -2.4081) (-1.0222, -1.7638) (-1.0679, -0.9976) (-1.1169, -0.2713) (-1.1684, 0.4156) (-1.2212, 1.065) (-1.2733, 1.6815) (-1.3218, 2.2727) (-1.3636, 2.8473) (-1.3954, 3.4143) (-1.4149, 3.9813) (-1.4204, 4.5534) (-1.4115, 5.1335) (-1.3928, 5.6049) (-1.3724, 5.9626) (-1.356, 6.203) (-1.3471, 6.3237) knots 0 0 0 0 0 0 0.066667 0.133333 0.2 0.266667 0.333333 0.4 0.466667 0.533333 0.6 0.666667 0.733333 0.8 0.866667 0.933333 1 1 1 1 1 1
  spline S7 degree 5 poles (-1.3471, 6.3237) (-1.3504, 6.3307) (-1.3558, 6.3452) (-1.3601, 6.3682) (-1.3582, 6.4012) (-1.3433, 6.4468) (-1.317, 6.4976) (-1.2807, 6.5552) (-1.2355, 6.6218) (-1.1802, 6.7004) (-1.1119, 6.794) (-1.0265, 6.9056) (-0.921, 7.037) (-0.7941, 7.1886) (-0.6473, 7.3587) (-0.484, 7.5444) (-0.3086, 7.7418) (-0.1261, 7.9465) (0.059, 8.1541) (0.2432, 8.3606) (0.4248, 8.5631) (0.6039, 8.7593) (0.7816, 8.9479) (0.9599, 9.1281) (1.1411, 9.2998) (1.3274, 9.463) (1.5206, 9.618) (1.7217, 9.7654) (1.9305, 9.9058) (2.1469, 10.04) (2.3701, 10.1692) (2.5996, 10.2948) (2.8349, 10.4189) (3.0763, 10.5438) (3.3244, 10.6725) (3.5802, 10.8079) (3.8446, 10.9529) (4.1178, 11.1093) (4.399, 11.2781) (4.6859, 11.4584) (4.9747, 11.6479) (5.259, 11.8414) (5.5303, 12.0315) (5.7794, 12.2096) (5.9978, 12.3676) (6.1793, 12.4985) (6.3215, 12.5984) (6.4267, 12.6669) (6.5049, 12.7096) (6.5715, 12.7372) (6.6402, 12.7622) (6.7156, 12.7955) (6.786, 12.8433) (6.8348, 12.9072) (6.8516, 12.984) (6.8452, 13.0661) (6.839, 13.1431) (6.8611, 13.2044) (6.934, 13.2417) (7.0721, 13.2497) (7.2841, 13.2251) (7.5161, 13.1781) (7.7259, 13.1273) (7.8816, 13.0866) (7.9635, 13.0644) knots 0 0 0 0 0 0 0.01666667 0.03333333 0.05 0.06666667 0.08333333 0.1 0.11666667 0.13333333 0.15 0.16666667 0.18333333 0.2 0.21666667 0.23333333 0.25 0.26666667 0.28333333 0.3 0.31666667 0.33333333 0.35 0.36666667 0.38333333 0.4 0.41666667 0.43333333 0.45 0.46666667 0.48333333 0.5 0.51666667 0.53333333 0.55 0.56666667 0.58333333 0.6 0.61666667 0.63333333 0.65 0.66666667 0.68333333 0.7 0.71666667 0.73333333 0.75 0.76666667 0.78333333 0.8 0.81666667 0.83333333 0.85 0.86666667 0.88333333 0.9 0.91666667 0.93333333 0.95 0.96666667 0.98333333 1 1 1 1 1 1
  spline S8 degree 5 poles (7.9635, 13.0644) (7.9956, 13.0561) (8.061, 13.0367) (8.163, 13.0002) (8.3067, 12.9362) (8.4991, 12.8312) (8.7035, 12.7023) (8.9189, 12.5521) (9.143, 12.3852) (9.3736, 12.2072) (9.609, 12.0234) (9.849, 11.8377) (10.0959, 11.6513) (10.3557, 11.4612) (10.6364, 11.2614) (10.9462, 11.0452) (11.2916, 10.8063) (11.6755, 10.5416) (12.0954, 10.252) (12.5409, 9.9451) (12.9948, 9.6346) (13.4363, 9.3365) (13.844, 9.0674) (14.1987, 8.8408) (14.4865, 8.6651) (14.7013, 8.5408) (14.8492, 8.4569) (14.9473, 8.3915) (15.0167, 8.3198) (15.0774, 8.2191) (15.1412, 8.0758) (15.1995, 7.922) (15.2482, 7.7837) (15.2829, 7.6813) (15.3008, 7.6276) knots 0 0 0 0 0 0 0.033333 0.066667 0.1 0.133333 0.166667 0.2 0.233333 0.266667 0.3 0.333333 0.366667 0.4 0.433333 0.466667 0.5 0.533333 0.566667 0.6 0.633333 0.666667 0.7 0.733333 0.766667 0.8 0.833333 0.866667 0.9 0.933333 0.966667 1 1 1 1 1 1
  spline S9 degree 5 poles (15.3008, 7.6276) (15.2991, 7.6275) (15.297, 7.6225) (15.2972, 7.6005) (15.3046, 7.5423) (15.3247, 7.4263) (15.3532, 7.283) (15.385, 7.1429) (15.4147, 7.0363) (15.4379, 6.9826) (15.4532, 6.9726) (15.4622, 6.9737) (15.467, 6.953) (15.4694, 6.8914) (15.4706, 6.7792) (15.4716, 6.6128) (15.4736, 6.3918) (15.4776, 6.1191) (15.4844, 5.8) (15.4946, 5.4413) (15.5085, 5.0508) (15.5261, 4.6366) (15.547, 4.2066) (15.5707, 3.7685) (15.5963, 3.3288) (15.6231, 2.8936) (15.6503, 2.4671) (15.6772, 2.0523) (15.7033, 1.6502) (15.7284, 1.2593) (15.7525, 0.8761) (15.776, 0.4951) (15.7993, 0.1104) (15.8229, -0.2839) (15.8471, -0.6927) (15.8722, -1.119) (15.898, -1.5632) (15.9242, -2.0222) (15.9497, -2.4883) (15.9732, -2.9505) (15.9931, -3.3955) (16.0077, -3.8085) (16.0152, -4.1749) (16.0142, -4.481) (16.0032, -4.7151) (15.9812, -4.8688) (15.9545, -4.9241) (15.9293, -4.9271) (15.9101, -4.9119) (15.9, -4.9) knots 0 0 0 0 0 0 0.022222 0.044444 0.066667 0.088889 0.111111 0.133333 0.155556 0.177778 0.2 0.222222 0.244444 0.266667 0.288889 0.311111 0.333333 0.355556 0.377778 0.4 0.422222 0.444444 0.466667 0.488889 0.511111 0.533333 0.555556 0.577778 0.6 0.622222 0.644444 0.666667 0.688889 0.711111 0.733333 0.755556 0.777778 0.8 0.822222 0.844444 0.866667 0.888889 0.911111 0.933333 0.955556 0.977778 1 1 1 1 1 1
  spline S10 degree 5 poles (21.4, 14.1) (21.3683, 14.0811) (21.298, 14.0386) (21.1718, 13.9602) (20.9622, 13.8266) (20.6324, 13.6119) (20.2393, 13.3516) (19.7914, 13.0503) (19.3033, 12.7154) (18.7966, 12.3583) (18.3026, 11.9953) (17.8598, 11.6466) (17.5036, 11.3334) (17.2584, 11.0748) (17.1279, 10.8843) (17.0875, 10.7674) (17.0726, 10.718) (16.9796, 10.7165) (16.7374, 10.7374) (16.3697, 10.7561) (15.9579, 10.7528) (15.6003, 10.7165) (15.374, 10.6492) (15.2922, 10.571) (15.2739, 10.5211) (15.2173, 10.5366) (15.079, 10.6264) (14.8649, 10.7781) (14.6037, 10.9699) (14.3229, 11.1825) (14.0345, 11.4056) (13.7416, 11.6347) (13.4403, 11.8692) (13.1233, 12.1107) (12.7828, 12.3609) (12.4138, 12.6198) (12.0152, 12.885) (11.5893, 13.153) (11.1418, 13.4195) (10.6813, 13.68) (10.2196, 13.9305) (9.771, 14.1682) (9.3528, 14.392) (8.984, 14.6028) (8.6813, 14.8022) (8.4553, 14.9913) (8.3067, 15.1693) (8.223, 15.333) (8.1731, 15.4741) (8.1189, 15.5884) (8.0313, 15.6861) (7.906, 15.8042) (7.7577, 15.9954) (7.6095, 16.3122) (7.4848, 16.7934) (7.3967, 17.4484) (7.3495, 18.2609) (7.3406, 19.1957) (7.3626, 20.2036) (7.4049, 21.2277) (7.4558, 22.2084) (7.5045, 23.09) (7.543, 23.8254) (7.5676, 24.3825) (7.5816, 24.7498) (7.5963, 24.9412) (7.634, 25.0043) (7.7219, 25.0027) (7.8829, 24.9923) (8.1319, 25.0086) (8.4778, 25.0734) (8.8354, 25.1727) (9.1497, 25.2753) (9.3798, 25.3564) (9.5, 25.4) knots 0 0 0 0 0 0 0.01428571 0.02857143 0.04285714 0.05714286 0.07142857 0.08571429 0.1 0.11428571 0.12857143 0.14285714 0.15714286 0.17142857 0.18571429 0.2 0.21428571 0.22857143 0.24285714 0.25714286 0.27142857 0.28571429 0.3 0.31428571 0.32857143 0.34285714 0.35714286 0.37142857 0.38571429 0.4 0.41428571 0.42857143 0.44285714 0.45714286 0.47142857 0.48571429 0.5 0.51428571 0.52857143 0.54285714 0.55714286 0.57142857 0.58571429 0.6 0.61428571 0.62857143 0.64285714 0.65714286 0.67142857 0.68571429 0.7 0.71428571 0.72857143 0.74285714 0.75714286 0.77142857 0.78571429 0.8 0.81428571 0.82857143 0.84285714 0.85714286 0.87142857 0.88571429 0.9 0.91428571 0.92857143 0.94285714 0.95714286 0.97142857 0.98571429 1 1 1 1 1 1
  spline S11 degree 5 poles (9.5, 25.4) (9.5682, 25.389) (9.7075, 25.3621) (9.9256, 25.3073) (10.2345, 25.2054) (10.65, 25.0305) (11.0914, 24.8113) (11.5517, 24.555) (12.0186, 24.2738) (12.4786, 23.9818) (12.9205, 23.6908) (13.3394, 23.4067) (13.7411, 23.1254) (14.1435, 22.8311) (14.5691, 22.5033) (15.0401, 22.1216) (15.573, 21.6714) (16.1711, 21.1497) (16.8243, 20.5664) (17.5134, 19.9401) (18.2128, 19.2948) (18.8943, 18.6576) (19.53, 18.0547) (20.0957, 17.509) (20.5747, 17.0365) (20.958, 16.6457) (21.1849, 16.4015) (21.31, 16.2572) (21.3733, 16.1783) (21.4, 16.1431) knots 0 0 0 0 0 0 0.04 0.08 0.12 0.16 0.2 0.24 0.28 0.32 0.36 0.4 0.44 0.48 0.52 0.56 0.6 0.64 0.68 0.72 0.76 0.8 0.84 0.88 0.92 0.96 1 1 1 1 1 1
  spline S12 degree 5 poles (5.1289, 15.8493) (4.8139, 15.6471) (4.1159, 15.1954) (3.1044, 14.5271) (1.8974, 13.6984) (0.6589, 12.7881) (-0.3265, 11.9868) (-1.0188, 11.3342) (-1.4487, 10.8249) (-1.663, 10.4507) (-1.7287, 10.1995) (-1.7346, 10.055) (-1.7999, 9.9953) (-2.0569, 9.9941) (-2.5363, 10.0267) (-3.1314, 10.0744) (-3.6919, 10.1273) (-4.0859, 10.1869) (-4.2861, 10.2704) (-4.4118, 10.4099) (-4.623, 10.6354) (-5.0182, 10.9564) (-5.6146, 11.3604) (-6.3786, 11.8225) (-7.241, 12.3107) (-8.1184, 12.7934) (-8.9301, 13.245) (-9.6214, 13.6542) (-10.1717, 14.0266) (-10.5835, 14.3785) (-10.8757, 14.7336) (-11.0751, 15.1184) (-11.2079, 15.5577) (-11.2946, 16.071) (-11.3515, 16.6726) (-11.3912, 17.3696) (-11.4234, 18.1617) (-11.4558, 19.0393) (-11.4943, 19.9843) (-11.5429, 20.9729) (-11.6034, 21.9778) (-11.6752, 22.9706) (-11.7553, 23.9247) (-11.8378, 24.817) (-11.914, 25.6311) (-11.9718, 26.3592) (-11.9975, 27.0008) (-11.9768, 27.5599) (-11.8966, 28.0428) (-11.7459, 28.4563) (-11.518, 28.8049) (-11.2714, 29.0338) (-11.0499, 29.1777) (-10.886, 29.2613) (-10.8, 29.3) knots 0.004459 0.004459 0.004459 0.004459 0.004459 0.004459 0.02 0.04 0.06 0.08 0.1 0.12 0.14 0.16 0.18 0.2 0.22 0.24 0.26 0.28 0.3 0.32 0.34 0.36 0.38 0.4 0.42 0.44 0.46 0.48 0.5 0.52 0.54 0.56 0.58 0.6 0.62 0.64 0.66 0.68 0.7 0.72 0.74 0.76 0.78 0.8 0.82 0.84 0.86 0.88 0.9 0.92 0.94 0.96 0.98 1 1 1 1 1 1
  line L4 (-38.2, -26) -> (19.4, -26)
  line L5 (21.4, -24) -> (21.4, 23.2)
  arc A18 (19.4, -26) -> (21.4, -24) centre (19.4, -24) ccw
  arc A19 (21.4, 23.2) -> (19.4, 25.2) centre (19.4, 23.2) ccw
  line L6 (19.4, 25.2) -> (-38.2, 25.2)
  arc A20 (-38.2, 25.2) -> (-40.2, 23.2) centre (-38.2, 23.2) ccw
  line L7 (-40.2, 23.2) -> (-40.2, -24)
  arc A21 (-40.2, -24) -> (-38.2, -26) centre (-38.2, -24) ccw
  spline S13 degree 5 poles (5.5887, 16.6908) (5.5887, 16.7205) (5.5887, 16.8925) (5.5887, 17.2124) (5.5887, 17.6925) (5.5887, 18.3528) (5.5887, 19.1858) (5.5887, 20.0706) (5.5887, 21.0069) (5.5887, 21.9912) (5.5887, 23.019) (5.5887, 23.873) (5.5887, 24.5302) (5.5887, 24.9755) (5.5887, 25.2) knots 0.079102 0.079102 0.079102 0.079102 0.079102 0.079102 0.1 0.2 0.3 0.4 0.5 0.6 0.7 0.8 0.9 1 1 1 1 1 1
  arc A22 (5.1289, 15.8493) -> (5.5887, 16.6908) centre (4.5887, 16.6908) ccw
  spline S14 degree 5 poles (-13.9645, 25.2) (-13.9621, 24.9666) (-13.9564, 24.5026) (-13.9457, 23.8157) (-13.9269, 22.9179) (-13.8954, 21.828) (-13.8551, 20.7737) (-13.8053, 19.7584) (-13.7451, 18.7846) (-13.6748, 17.852) (-13.5949, 16.958) (-13.5239, 16.2713) (-13.467, 15.7714) (-13.4274, 15.4448) (-13.4072, 15.2831) knots 0 0 0 0 0 0 0.1 0.2 0.3 0.4 0.5 0.6 0.7 0.8 0.9 1 1 1 1 1 1
  spline S15 degree 5 poles (-13.4072, 15.2831) (-13.3961, 15.2634) (-13.379, 15.2233) (-13.3681, 15.1617) (-13.3833, 15.0765) (-13.4513, 14.9644) (-13.5665, 14.8451) (-13.7252, 14.7154) (-13.922, 14.5711) (-14.1521, 14.4075) (-14.4113, 14.2202) (-14.698, 14.0059) (-15.0128, 13.7624) (-15.3577, 13.4888) (-15.7347, 13.186) (-16.1447, 12.8562) (-16.5867, 12.5032) (-17.0563, 12.133) (-17.5447, 11.753) (-18.0375, 11.3731) (-18.5167, 11.0042) (-18.9635, 10.6576) (-19.3598, 10.3435) (-19.6914, 10.0706) (-19.95, 9.8449) (-20.1355, 9.6687) (-20.2587, 9.5394) (-20.3429, 9.4488) (-20.4161, 9.3864) (-20.5045, 9.3416) (-20.6238, 9.3071) (-20.7808, 9.2783) (-20.9767, 9.2528) (-21.2106, 9.2293) (-21.4821, 9.2067) (-21.7907, 9.1845) (-22.0671, 9.1668) (-22.2908, 9.1536) (-22.4473, 9.1448) (-22.5273, 9.1404) knots 0 0 0 0 0 0 0.028571 0.057143 0.085714 0.114286 0.142857 0.171429 0.2 0.228571 0.257143 0.285714 0.314286 0.342857 0.371429 0.4 0.428571 0.457143 0.485714 0.514286 0.542857 0.571429 0.6 0.628571 0.657143 0.685714 0.714286 0.742857 0.771429 0.8 0.828571 0.857143 0.885714 0.914286 0.942857 0.971429 1 1 1 1 1 1
  spline S16 degree 5 poles (-22.5273, 9.1404) (-22.5348, 9.1323) (-22.5511, 9.1197) (-22.5799, 9.1119) (-22.6269, 9.1238) (-22.7042, 9.176) (-22.8132, 9.2668) (-22.9717, 9.3968) (-23.1953, 9.5654) (-23.4912, 9.7684) (-23.8512, 9.9975) (-24.2551, 10.241) (-24.6763, 10.4859) (-25.0858, 10.7199) (-25.4574, 10.9327) (-25.7724, 11.1183) (-26.0241, 11.2764) (-26.2237, 11.4147) (-26.3991, 11.5484) (-26.585, 11.6946) (-26.8143, 11.8688) (-27.1101, 12.0804) (-27.4756, 12.3282) (-27.8915, 12.5988) (-28.3256, 12.8726) (-28.7394, 13.1277) (-29.0961, 13.3448) (-29.3677, 13.5109) (-29.5422, 13.6244) (-29.6325, 13.6999) (-29.6798, 13.77) (-29.7301, 13.8674) (-29.8107, 14.0068) (-29.9151, 14.1739) (-30.0223, 14.3438) (-30.108, 14.4926) (-30.1621, 14.6154) (-30.191, 14.7262) (-30.2073, 14.8461) (-30.2222, 14.9919) (-30.2404, 15.1712) (-30.2635, 15.3864) (-30.2909, 15.6372) (-30.3214, 15.9239) (-30.3544, 16.2477) (-30.3892, 16.6103) (-30.4249, 17.0127) (-30.4609, 17.4551) (-30.4965, 17.9358) (-30.5306, 18.4505) (-30.5623, 18.992) (-30.5903, 19.5505) (-30.6135, 20.1146) (-30.6307, 20.6722) (-30.6408, 21.2115) (-30.6428, 21.7216) (-30.636, 22.1935) (-30.6201, 22.6211) (-30.5948, 23.0018) (-30.5605, 23.3375) (-30.5178, 23.6339) (-30.4676, 23.8985) (-30.4107, 24.1397) (-30.348, 24.3654) (-30.2799, 24.5816) (-30.207, 24.792) (-30.1449, 24.957) (-30.0963, 25.0791) (-30.0629, 25.1598) (-30.046, 25.2) knots 0 0 0 0 0 0 0.01538462 0.03076923 0.04615385 0.06153846 0.07692308 0.09230769 0.10769231 0.12307692 0.13846154 0.15384615 0.16923077 0.18461538 0.2 0.21538462 0.23076923 0.24615385 0.26153846 0.27692308 0.29230769 0.30769231 0.32307692 0.33846154 0.35384615 0.36923077 0.38461538 0.4 0.41538462 0.43076923 0.44615385 0.46153846 0.47692308 0.49230769 0.50769231 0.52307692 0.53846154 0.55384615 0.56923077 0.58461538 0.6 0.61538462 0.63076923 0.64615385 0.66153846 0.67692308 0.69230769 0.70769231 0.72307692 0.73846154 0.75384615 0.76923077 0.78461538 0.8 0.81538462 0.83076923 0.84615385 0.86153846 0.87692308 0.89230769 0.90769231 0.92307692 0.93846154 0.95384615 0.96923077 0.98461538 1 1 1 1 1 1
  spline S17 degree 5 poles (-35.8, 25.2) (-35.8577, 25.1567) (-35.9759, 25.0681) (-36.1615, 24.9288) (-36.4259, 24.7306) (-36.7863, 24.4603) (-37.1789, 24.1658) (-37.6055, 23.8458) (-38.066, 23.5005) (-38.5578, 23.1317) (-39.078, 22.7415) (-39.5148, 22.4139) (-39.8533, 22.16) (-40.0836, 21.9873) (-40.2, 21.9) knots 0 0 0 0 0 0 0.1 0.2 0.3 0.4 0.5 0.6 0.7 0.8 0.9 1 1 1 1 1 1